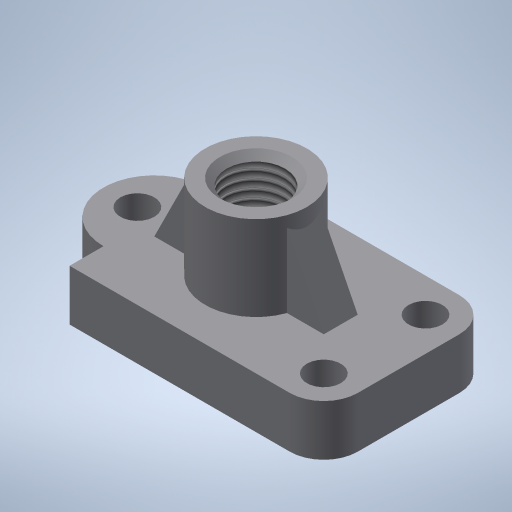
# Autodesk Inventor part: Основание
Saved by Autodesk Inventor 2023.2 (Build 272271030, 271C)
## iProperties
Created: 2017-03-09
Part Number: Основание
Material: Типовые
Document SubType Name: Modeling
Designer: Cтас
Density: 1 g/cm^3
Appearance: По умолчанию
Author: Cтас
Autodesk Inventor part; units mm, degrees
ref_plane "YZ Plane" through (0, 0, 0) normal (1, 0, 0) x (0, 1, 0)
ref_plane "XZ Plane" through (0, 0, 0) normal (0, 1, 0) x (-1, 0, 0)
ref_plane "XY Plane" through (0, 0, 0) normal (0, 0, 1) x (1, 0, 0)
sketch "Эскиз1" plane through (0, 0, 0) normal (0, 0, 1) x (1, 0, 0)
  line L0 (-30, 25) -> (35, 25)
  line L1 (45, 15) -> (45, -15)
  line L2 (35, -25) -> (-30, -25)
  line L3 (-63.4142, 0) -> (65.4853, 0) projected
  line L4 (0, -37.8995) -> (0, 37.8995) projected
  arc A0 (45, 15) -> (35, 25) centre (35, 15) ccw
  arc A1 (35, -25) -> (45, -15) centre (35, -15) ccw
  circle A2 centre (35, 15) radius 5
  circle A3 centre (35, -15) radius 5
  circle A4 centre (-35, 0) radius 5
  line L5 (-30, -25) -> (-30, -15)
  line L6 (-30, 15) -> (-30, 25)
  arc A5 (-30, 15) -> (-30, -15) centre (-30, 0) ccw
  line L7 (-45, 22.4423) -> (-45, -16.9237) construction
  point P0 (0, 0)
  dimension "d1" = 50
  dimension "d2" = 10
  dimension "d3" = 10
  dimension "d4" = 10
  dimension "d5" = 30
  dimension "d6" = 10
  dimension "d7" = 35
  dimension "d8" = 35
  dimension "d11" = 75
  dimension "d46" = 30
  dimension "d47" = 90
  constraints: 12 end point, 6 centre point, 6 point on circle, 4 parallel, 4 symmetric about line, 3 tangent, 2 point on line, 1 horizontal, 1 perpendicular, 4 other
  measures "d1" distance between parallel lines of L2 L0
  measures "d2" radius of A0
  measures "d3" diameter of A2
  measures "d4" distance from line of L1 A2.centre
  measures "d5" distance of A2.centre A3.centre
  measures "d6" diameter of A4
  measures "d7" distance from line of L4 A4.centre
  measures "d8" distance from line of L4 A0.centre
  measures "d11" distance between parallel lines of L1 L5
  measures "d46" diameter of A5
  measures "d47" distance between parallel lines of L1 L7
extrude "Выдавливание1" add sketch "Эскиз1" along normal blind 15 contours L0 L4 L3 A4 A5 L6 | L0 A0 L1 L3 L4 | L4 L2 L5 A5 L3 A4 | L3 L1 A1 L2 L4
sketch "Эскиз2" plane through (0, 0, 15) normal (0, 0, 1) x (1, 0, 0)
  circle A0 centre (0, 0) radius 15
  dimension "d14" = 30
  constraints: 1 centre point, 1 coincident
  measures "d14" diameter of A0
extrude "Выдавливание2" add sketch "Эскиз2" along normal blind 25
hole "Отверстие1" at (0, 0, 40) direction (0, 0, -1) diameter 17.294 end through all thread size "M20x2.5" class "6H" standard "ANSI Metric M Profile"
chamfer "Фаска1" distance 2 angle 45 1 edges at (0, 8.647, 40)
sketch "Эскиз3" plane through (0, 0, 0) normal (0, 1, 0) x (-1, 0, 0)
  line L0 (30, 15) -> (30, 0) projected
  line L1 (30, 0) -> (8.647, 0) projected
  line L2 (8.647, 0) -> (8.647, 38) projected
  line L3 (8.647, 38) -> (10.647, 40) projected
  line L4 (10.647, 40) -> (15, 40) projected
  line L5 (15, 40) -> (15, 15) projected
  line L6 (15, 15) -> (30, 15) projected
  line L7 (-45, 0) -> (-45, 15) projected
  line L8 (-45, 15) -> (-15, 15) projected
  line L9 (-15, 15) -> (-15, 40) projected
  line L10 (-15, 40) -> (-10.647, 40) projected
  line L11 (-10.647, 40) -> (-8.647, 38) projected
  line L12 (-8.647, 38) -> (-8.647, 0) projected
  line L13 (-8.647, 0) -> (-45, 0) projected
  line L14 (45, 0) -> (40, 0) projected
  line L15 (40, 0) -> (40, 15) projected
  line L16 (40, 15) -> (45, 15) projected
  line L17 (-25, 15) -> (-15, 35)
  line L18 (15, 35) -> (25, 15)
  line L19 (0, -8) -> (0, 48) projected
  line L20 (45, 15) -> (45, 0) projected
  point P0 (0, 0)
  dimension "d29" = 5
  dimension "d30" = 5
  dimension "d31" = 50
  constraints: 4 end point, 4 point on line, 1 symmetric about line
  measures "d29" distance from line of L10 L17.end
  measures "d30" distance from line of L4 L18.start
  measures "d31" distance of L18.end L17.start
extrude "Ребро жесткости1" add sketch "Эскиз3" along normal mid plane 10 rib yes fills toward (19.9553, 24.9776) open curves L18
sketch "Эскиз4" plane through (0, 0, 0) normal (0, 1, 0) x (-1, 0, 0)
  line L0 (40, 0) -> (40, 15) projected
  line L1 (40, 15) -> (45, 15) projected
  line L2 (45, 0) -> (40, 0) projected
  line L3 (-15, 40) -> (-10.647, 40) projected
  line L4 (-10.647, 40) -> (-8.647, 38) projected
  line L5 (-8.647, 38) -> (-8.647, 0) projected
  line L6 (-8.647, 0) -> (-45, 0) projected
  line L7 (-45, 0) -> (-45, 15) projected
  line L8 (-45, 15) -> (-15, 15) projected
  line L9 (-15, 15) -> (-15, 40) projected
  line L10 (10.647, 40) -> (15, 40) projected
  line L11 (15, 40) -> (15, 35) projected
  line L12 (15, 35) -> (25, 15) projected
  line L13 (25, 15) -> (30, 15) projected
  line L14 (30, 15) -> (30, 0) projected
  line L15 (30, 0) -> (8.647, 0) projected
  line L16 (8.647, 0) -> (8.647, 38) projected
  line L17 (8.647, 38) -> (10.647, 40) projected
  line L18 (-25, 15) -> (-15, 35)
  line L19 (45, 15) -> (45, 0) projected
  point P0 (0, 0)
  dimension "d38" = 5
  dimension "d39" = 50
  constraints: 2 end point, 2 point on line
  measures "d38" distance from line of L3 L18.end
  measures "d39" distance of L18.start L12.end
extrude "Ребро жесткости2" add sketch "Эскиз4" along normal mid plane 10 rib yes fills toward (-19.9553, 24.9776) open curves L18
